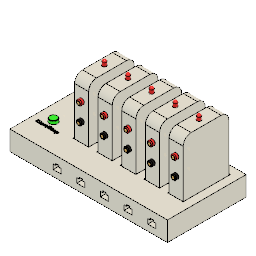
Messbox v3 (Autodesk Fusion 360 design; units mm, degrees)
Autodesk Fusion 360 part; units mm, degrees
sketch "Skizze1" plane through (0, 0, 0) normal (0, 1, 0) x (1, 0, 0)
  line L0 (0, 0) -> (200, 0)
  line L1 (200, 0) -> (200, -100)
  line L2 (200, -100) -> (0, -100)
  line L3 (0, -100) -> (0, 0)
  dimension "d1" = 200
  dimension "d2" = 100
  constraint horizontal L0
  constraint vertical L1
  constraint horizontal L2
  constraint vertical L3
  constraint coincident L0.start L3.end
  measures "d1" distance of L0.start L0.end
  measures "d2" distance of L0.end L1.end
  measures "d91" distance of L0.start
extrude "Extrusion1" add sketch "Skizze1" along normal blind 25
sketch "Skizze2" plane through (0, 25, 0) normal (0, 1, 0) x (-1, 0, 0)
  line L0 (0, 100) -> (-200, 100)
  line L1 (-200, 100) -> (-200, 0)
  line L2 (-200, 0) -> (0, 0)
  line L3 (0, 0) -> (0, 100)
  line L4 (-170, 10) -> (-190, 10)
  line L5 (-190, 10) -> (-190, 70)
  line L6 (-190, 70) -> (-170, 70)
  line L7 (-170, 70) -> (-170, 10)
  line L8 (-140, 10) -> (-160, 10)
  line L9 (-160, 10) -> (-160, 70)
  line L10 (-160, 70) -> (-140, 70)
  line L11 (-140, 70) -> (-140, 10)
  line L12 (-110, 10) -> (-130, 10)
  line L13 (-130, 10) -> (-130, 70)
  line L14 (-130, 70) -> (-110, 70)
  line L15 (-110, 70) -> (-110, 10)
  line L16 (-80, 10) -> (-100, 10)
  line L17 (-100, 10) -> (-100, 70)
  line L18 (-100, 70) -> (-80, 70)
  line L19 (-80, 70) -> (-80, 10)
  line L20 (-100, 10) -> (-110, 10) construction
  line L21 (-130, 10) -> (-140, 10) construction
  line L22 (-160, 10) -> (-170, 10) construction
  line L23 (-70, 10) -> (-50, 10)
  line L24 (-50, 10) -> (-50, 70)
  line L25 (-50, 70) -> (-70, 70)
  line L26 (-70, 70) -> (-70, 10)
  line L27 (-70, 10) -> (-80, 10) construction
  dimension "d5" = 10
  dimension "d6" = 10
  dimension "d8" = 20
  dimension "d38" = 50
  dimension "d162" = 60
  constraint horizontal L4
  constraint vertical L5
  constraint horizontal L6
  constraint vertical L7
  constraint horizontal L8
  constraint vertical L9
  constraint horizontal L10
  constraint vertical L11
  constraint horizontal L12
  constraint vertical L13
  constraint horizontal L14
  constraint vertical L15
  constraint horizontal L16
  constraint vertical L17
  constraint horizontal L18
  constraint vertical L19
  constraint equal L12 L16
  constraint equal L8 L12
  constraint equal L4 L8
  constraint perpendicular L15 L20
  constraint perpendicular L11 L21
  constraint perpendicular L7 L22
  constraint equal L20 L21
  constraint equal L21 L22
  constraint horizontal L13.end L17.end
  constraint horizontal L9.end L13.end
  constraint horizontal L5.end L9.end
  constraint horizontal L23
  constraint vertical L24
  constraint horizontal L25
  constraint vertical L26
  constraint horizontal L27
  constraint horizontal L17.end L25.end
  constraint equal L20 L27
  constraint equal L16 L23
  measures "d5" vertical distance of L1.end L4.end
  measures "d6" horizontal distance of L1.end L4.end
  measures "d8" distance of L4.start L4.end
  measures "d38" horizontal distance of L2.end L23.end
  measures "d162" distance of L4.end L5.end
extrude "Extrusion2" cut sketch "Skizze2" against normal blind 20 contours L4 L5 L6 L7 | L8 L9 L10 L11 | L12 L13 L14 L15 | L16 L17 L18 L19 | L23 L24 L25 L26
sketch "Skizze3" plane through (0, 5, 0) normal (0, 1, 0) x (-1, 0, 0)
  line L0 (-80, 70) -> (-100, 70)
  line L1 (-100, 70) -> (-100, 10)
  line L2 (-100, 10) -> (-80, 10)
  line L3 (-80, 10) -> (-80, 70)
  line L4 (-81, 11) -> (-99, 11)
  line L5 (-99, 11) -> (-99, 69)
  line L6 (-99, 69) -> (-81, 69)
  line L7 (-81, 69) -> (-81, 11)
  line L8 (-111, 11) -> (-129, 11)
  line L9 (-129, 11) -> (-129, 69)
  line L10 (-129, 69) -> (-111, 69)
  line L11 (-111, 69) -> (-111, 11)
  line L12 (-141, 11) -> (-159, 11)
  line L13 (-159, 11) -> (-159, 69)
  line L14 (-159, 69) -> (-141, 69)
  line L15 (-141, 69) -> (-141, 11)
  line L16 (-171, 11) -> (-189, 11)
  line L17 (-189, 11) -> (-189, 69)
  line L18 (-189, 69) -> (-171, 69)
  line L19 (-171, 69) -> (-171, 11)
  line L20 (-51, 11) -> (-69, 11)
  line L21 (-69, 11) -> (-69, 69)
  line L22 (-69, 69) -> (-51, 69)
  line L23 (-51, 69) -> (-51, 11)
  point P0 (-110, 10)
  point P1 (-130, 10)
  point P2 (-130, 70)
  point P3 (-110, 70)
  point P4 (-140, 10)
  point P5 (-160, 10)
  point P6 (-160, 70)
  point P7 (-140, 70)
  point P8 (-170, 10)
  point P9 (-190, 10)
  point P10 (-190, 70)
  point P11 (-70, 10)
  point P12 (-50, 70)
  dimension "d12" = 1
  dimension "d13" = 1
  dimension "d14" = 1
  dimension "d15" = 1
  dimension "d16" = 1
  dimension "d17" = 1
  dimension "d18" = 1
  dimension "d19" = 1
  dimension "d20" = 1
  dimension "d21" = 1
  dimension "d22" = 1
  dimension "d23" = 1
  dimension "d24" = 1
  dimension "d25" = 1
  dimension "d26" = 1
  dimension "d27" = 1
  dimension "d39" = 1
  dimension "d40" = 1
  dimension "d41" = 1
  dimension "d42" = 1
  constraint horizontal L4
  constraint vertical L5
  constraint horizontal L6
  constraint vertical L7
  constraint horizontal L8
  constraint vertical L9
  constraint horizontal L10
  constraint vertical L11
  constraint horizontal L12
  constraint vertical L13
  constraint horizontal L14
  constraint vertical L15
  constraint horizontal L16
  constraint vertical L17
  constraint horizontal L18
  constraint vertical L19
  constraint horizontal L20
  constraint vertical L21
  constraint horizontal L22
  constraint vertical L23
  measures "d12" horizontal distance of L2.end L4.start
  measures "d13" horizontal distance of L1.end L4.end
  measures "d14" vertical distance of L1.end L4.end
  measures "d15" vertical distance of L0.end L5.end
  measures "d16" horizontal distance of L8.start P0
  measures "d17" vertical distance of L8.end P1
  measures "d18" horizontal distance of L9.end P2
  measures "d19" vertical distance of L10.end P3
  measures "d20" horizontal distance of L12.start P4
  measures "d21" vertical distance of L12.end P5
  measures "d22" horizontal distance of L13.end P6
  measures "d23" vertical distance of L14.end P7
  measures "d24" horizontal distance of L16.start P8
  measures "d25" horizontal distance of L16.end P9
  measures "d26" vertical distance of L17.end P10
  measures "d27" vertical distance of L16.end P9
  measures "d39" horizontal distance of L20.end P11
  measures "d40" vertical distance of L20.end P11
  measures "d41" vertical distance of L22.end P12
  measures "d42" horizontal distance of L22.end P12
extrude "Extrusion3" add sketch "Skizze3" along normal blind 90 contours L4 L5 L6 L7 | L8 L9 L10 L11 | L12 L13 L14 L15 | L16 L17 L18 L19 | L20 L21 L22 L23
fillet "Abrundung1" radius 10 8 edges at (90, 95, 69) (120, 95, 69) (120, 95, 11) (90, 95, 11) (150, 95, 11) (180, 95, 11) (180, 95, 69) (150, 95, 69)
fillet "Abrundung3" radius 10 2 edges at (60, 95, 11) (60, 95, 69)
sketch "Skizze4" plane through (0, 95, 0) normal (0, 1, 0) x (-1, 0, 0)
  line L0 (-99, 21) -> (-81, 21)
  line L1 (-81, 21) -> (-81, 59)
  line L2 (-81, 59) -> (-99, 59)
  line L3 (-99, 59) -> (-99, 21)
  circle A0 centre (-90, 40) radius 2.5
  circle A1 centre (-120, 40) radius 2.5
  circle A2 centre (-150, 40) radius 2.5
  circle A3 centre (-180, 40) radius 2.5
  line L4 (-81, 21) -> (-99, 59) construction
  line L5 (-129, 21) -> (-111, 21) construction
  line L6 (-111, 21) -> (-111, 59) construction
  line L7 (-111, 59) -> (-129, 59) construction
  line L8 (-129, 59) -> (-129, 21) construction
  line L9 (-141, 59) -> (-159, 59) construction
  line L10 (-159, 59) -> (-159, 21) construction
  line L11 (-159, 21) -> (-141, 21) construction
  line L12 (-141, 21) -> (-141, 59) construction
  line L13 (-171, 59) -> (-189, 59) construction
  line L14 (-189, 59) -> (-189, 21) construction
  line L15 (-189, 21) -> (-171, 21) construction
  line L16 (-171, 21) -> (-171, 59) construction
  line L17 (-111, 21) -> (-129, 59) construction
  line L18 (-141, 21) -> (-159, 59) construction
  line L19 (-171, 21) -> (-189, 59) construction
  line L20 (-51, 59) -> (-69, 59)
  line L21 (-69, 59) -> (-69, 21)
  line L22 (-69, 21) -> (-51, 21)
  line L23 (-51, 21) -> (-51, 59)
  line L24 (-51, 21) -> (-69, 59) construction
  circle A4 centre (-60, 40) radius 2.5
  dimension "d31" = 5
  dimension "d32" = 5
  dimension "d33" = 5
  dimension "d34" = 5
  dimension "d44" = 5
  constraint coincident L0.end L1.start
  constraint coincident L2.end L3.start
  constraint coincident L5.end L6.start
  constraint coincident L7.end L8.start
  constraint coincident L11.end L12.start
  constraint coincident L9.end L10.start
  constraint coincident L15.end L16.start
  constraint coincident L13.end L14.start
  constraint midpoint A0.centre L4
  constraint midpoint A1.centre L17
  constraint midpoint A2.centre L18
  constraint midpoint A3.centre L19
  constraint coincident L22.end L23.start
  constraint coincident L20.end L21.start
  constraint midpoint L24 A4.centre
  measures "d31" diameter of A0
  measures "d32" diameter of A1
  measures "d33" diameter of A2
  measures "d34" diameter of A3
  measures "d44" diameter of A4
extrude "Extrusion4" add sketch "Skizze4" along normal blind 7 contours A0 | A1 | A2 | A3 | A4
fillet "Abrundung2" radius 2.5 4 edges at (92.3308, 102, 39.096) (122.3308, 102, 39.096) (152.3308, 102, 39.096) (182.3308, 102, 39.096)
fillet "Abrundung4" radius 2.5 1 edges at (62.3308, 102, 39.096)
sketch "Skizze5" plane through (0, 95, 0) normal (0, 1, 0) x (-1, 0, 0)
  circle A0 centre (-180, 40) radius 2.5
  line L0 (-171, 59) -> (-189, 59)
  line L1 (-189, 59) -> (-189, 21)
  line L2 (-189, 21) -> (-171, 21)
  line L3 (-171, 21) -> (-171, 59)
  circle A1 centre (-60, 40) radius 2.5
  circle A2 centre (-90, 40) radius 2.5
  circle A3 centre (-120, 40) radius 2.5
  circle A4 centre (-150, 40) radius 2.5
  circle A5 centre (-180, 40) radius 2.5
  circle A6 centre (-60, 40) radius 2.65
  circle A7 centre (-90, 40) radius 2.65
  circle A8 centre (-120, 40) radius 2.65
  circle A9 centre (-150, 40) radius 2.65
  circle A10 centre (-180, 40) radius 2.65
  dimension "d46" = 5.3
  dimension "d47" = 5.3
  dimension "d48" = 5.3
  dimension "d49" = 5.3
  dimension "d50" = 5.3
  constraint concentric A1 A6
  constraint concentric A2 A7
  constraint concentric A3 A8
  constraint concentric A4 A9
  constraint concentric A5 A10
  measures "d46" diameter of A6
  measures "d47" diameter of A7
  measures "d48" diameter of A8
  measures "d49" diameter of A9
  measures "d50" diameter of A10
sketch "Skizze6" plane through (0, 95, 0) normal (0, 1, 0) x (-1, 0, 0)
  circle A0 centre (-120, 40) radius 2.5
  line L0 (-129, 21) -> (-111, 21)
  line L1 (-111, 21) -> (-111, 59)
  line L2 (-111, 59) -> (-129, 59)
  line L3 (-129, 59) -> (-129, 21)
extrude "Extrusion5" cut sketch "Skizze5" against normal blind 5 contours A6 | A7 | A8 | A9 | A10
sketch "Skizze7" plane through (0, 0, 69) normal (0, 0, 1) x (1, 0, 0)
  line L0 (69, 85) -> (51, 85)
  line L1 (51, 85) -> (51, 5)
  line L2 (51, 5) -> (69, 5)
  line L3 (69, 5) -> (69, 85)
  circle A0 centre (60, 70) radius 3.5
  circle A1 centre (90, 70) radius 3.5
  circle A2 centre (120, 70) radius 3.5
  circle A3 centre (150, 70) radius 3.5
  circle A4 centre (180, 70) radius 3.5
  circle A5 centre (60, 48) radius 3.5
  circle A6 centre (90, 48) radius 3.5
  circle A7 centre (120, 48) radius 3.5
  circle A8 centre (150, 48) radius 3.5
  circle A9 centre (180, 48) radius 3.5
  line L4 (51, 85) -> (60, 70) construction
  line L5 (60, 70) -> (69, 85) construction
  line L6 (99, 85) -> (81, 85) construction
  line L7 (81, 85) -> (81, 5) construction
  line L8 (81, 5) -> (99, 5) construction
  line L9 (99, 5) -> (99, 85) construction
  line L10 (129, 85) -> (111, 85) construction
  line L11 (111, 85) -> (111, 5) construction
  line L12 (111, 5) -> (129, 5) construction
  line L13 (129, 5) -> (129, 85) construction
  line L14 (159, 85) -> (141, 85) construction
  line L15 (141, 85) -> (141, 5) construction
  line L16 (141, 5) -> (159, 5) construction
  line L17 (159, 5) -> (159, 85) construction
  line L18 (189, 85) -> (171, 85) construction
  line L19 (171, 85) -> (171, 5) construction
  line L20 (171, 5) -> (189, 5) construction
  line L21 (189, 5) -> (189, 85) construction
  line L22 (81, 85) -> (90, 70) construction
  line L23 (90, 70) -> (99, 85) construction
  line L24 (111, 85) -> (120, 70) construction
  line L25 (120, 70) -> (129, 85) construction
  line L26 (141, 85) -> (150, 70) construction
  line L27 (150, 70) -> (159, 85) construction
  line L28 (171, 85) -> (180, 70) construction
  line L29 (180, 70) -> (189, 85) construction
  dimension "d53" = 7
  dimension "d54" = 7
  dimension "d55" = 7
  dimension "d56" = 7
  dimension "d57" = 7
  dimension "d58" = 7
  dimension "d59" = 7
  dimension "d60" = 7
  dimension "d61" = 7
  dimension "d62" = 7
  dimension "d63" = 15
  dimension "d64" = 22
  constraint horizontal A0.centre A1.centre
  constraint horizontal A1.centre A2.centre
  constraint horizontal A2.centre A3.centre
  constraint horizontal A3.centre A4.centre
  constraint horizontal A5.centre A6.centre
  constraint horizontal A6.centre A7.centre
  constraint horizontal A8.centre A9.centre
  constraint horizontal A7.centre A8.centre
  constraint vertical A0.centre A5.centre
  constraint vertical A1.centre A6.centre
  constraint vertical A2.centre A7.centre
  constraint vertical A3.centre A8.centre
  constraint vertical A4.centre A9.centre
  constraint coincident L0.end L1.start
  constraint coincident A0.centre L4.end
  constraint coincident L0.start L3.end
  constraint coincident L6.end L7.start
  constraint coincident A1.centre L22.end
  constraint coincident L6.start L9.end
  constraint coincident L10.end L11.start
  constraint coincident A2.centre L24.end
  constraint coincident L10.start L13.end
  constraint coincident L14.end L15.start
  constraint coincident A3.centre L26.end
  constraint coincident L14.start L17.end
  constraint coincident L18.end L19.start
  constraint coincident A4.centre L28.end
  constraint coincident L18.start L21.end
  constraint equal L4 L5
  constraint equal L22 L23
  constraint equal L24 L25
  constraint equal L26 L27
  constraint equal L28 L29
  measures "d53" diameter of A0
  measures "d54" diameter of A1
  measures "d55" diameter of A2
  measures "d56" diameter of A3
  measures "d57" diameter of A4
  measures "d58" diameter of A5
  measures "d59" diameter of A6
  measures "d60" diameter of A7
  measures "d61" diameter of A8
  measures "d62" diameter of A9
  measures "d63" vertical distance of L0.end A0.centre
  measures "d64" distance of A0.centre A5.centre
extrude "Extrusion6" add sketch "Skizze7" along normal blind 4 contours A0 | A1 | A2 | A3 | A4 | A5 | A6 | A7 | A8 | A9
sketch "Skizze8" plane through (0, 0, 73) normal (0, 0, 1) x (1, 0, 0)
  circle A0 centre (60, 70) radius 3.5
  circle A1 centre (120, 48) radius 3.5
  circle A2 centre (150, 48) radius 3.5
  circle A3 centre (150, 70) radius 3.5
  circle A4 centre (120, 70) radius 3.5
  circle A5 centre (90, 48) radius 3.5
  circle A6 centre (90, 70) radius 3.5
  circle A7 centre (60, 48) radius 3.5
  circle A8 centre (60, 70) radius 3.5
  circle A9 centre (180, 70) radius 3.5
  circle A10 centre (180, 48) radius 3.5
  circle A11 centre (60, 70) radius 2
  circle A12 centre (60, 48) radius 2
  circle A13 centre (90, 70) radius 2
  circle A14 centre (90, 48) radius 2
  circle A15 centre (120, 70) radius 2
  circle A16 centre (120, 48) radius 2
  circle A17 centre (150, 70) radius 2
  circle A18 centre (150, 48) radius 2
  circle A19 centre (180, 70) radius 2
  circle A20 centre (180, 48) radius 2
  point P0 (176.5, 70)
  dimension "d67" = 4
  dimension "d68" = 4
  dimension "d69" = 4
  dimension "d70" = 4
  dimension "d71" = 4
  dimension "d72" = 4
  dimension "d73" = 4
  dimension "d74" = 4
  dimension "d75" = 4
  dimension "d76" = 4
  constraint concentric A0 A11
  constraint concentric A7 A12
  constraint concentric A6 A13
  constraint concentric A5 A14
  constraint concentric A4 A15
  constraint concentric A1 A16
  constraint concentric A3 A17
  constraint concentric A2 A18
  constraint concentric A9 A19
  constraint concentric A10 A20
  measures "d67" diameter of A11
  measures "d68" diameter of A12
  measures "d69" diameter of A13
  measures "d70" diameter of A14
  measures "d71" diameter of A15
  measures "d72" diameter of A16
  measures "d73" diameter of A17
  measures "d74" diameter of A18
  measures "d75" diameter of A19
  measures "d76" diameter of A20
extrude "Extrusion7" cut sketch "Skizze8" against normal blind 20 contours A11 | A12 | A13 | A14 | A15 | A16 | A17 | A18 | A19 | A20
fillet "Abrundung5" radius 1 10 edges at (56.7369, 68.7343, 73) (56.7369, 46.7343, 73) (86.7369, 46.7343, 73) (86.7369, 68.7343, 73) (116.7369, 68.7343, 73) (116.7369, 46.7343, 73) (146.7369, 68.7343, 73) (146.7369, 46.7343, 73) (176.7369, 68.7343, 73) (176.7369, 46.7343, 73)
sketch "Skizze9" plane through (0, 0, 0) normal (-1, 0, 0) x (0, 0, 1)
  line L0 (0, 0) -> (100, 0)
  line L1 (100, 0) -> (100, 25)
  line L2 (100, 25) -> (0, 25)
  line L3 (0, 25) -> (0, 0)
  line L4 (25.4, 8.1539) -> (34.4, 8.1539)
  line L5 (34.4, 8.1539) -> (34.4, 4.1539)
  line L6 (34.4, 4.1539) -> (25.4, 4.1539)
  line L7 (25.4, 4.1539) -> (25.4, 8.1539)
  line L8 (54.9, 7.1539) -> (62.9, 7.1539)
  line L9 (62.9, 7.1539) -> (62.9, 4.1539)
  line L10 (62.9, 4.1539) -> (54.9, 4.1539)
  line L11 (54.9, 4.1539) -> (54.9, 7.1539)
  line L12 (67.5, 7.1539) -> (75.5, 7.1539)
  line L13 (75.5, 7.1539) -> (75.5, 4.1539)
  line L14 (75.5, 4.1539) -> (67.5, 4.1539)
  line L15 (67.5, 4.1539) -> (67.5, 7.1539)
  line L16 (0, 0) -> (17.5, 0) construction
  line L17 (82.5, 0) -> (100, 0) construction
  point P0 (29.9, 4.1539)
  point P1 (58.9, 4.1539)
  point P2 (71.5, 4.1539)
  point P3 (17.5, 0)
  point P4 (82.5, 0)
  dimension "d80" = 9
  dimension "d81" = 4
  dimension "d82" = 8
  dimension "d83" = 8
  dimension "d84" = 3
  dimension "d85" = 3
  dimension "d88" = 12.4
  dimension "d90" = 41.4
  dimension "d91" = 54
  dimension "d92" = 65
  constraint horizontal L4
  constraint vertical L5
  constraint horizontal L6
  constraint vertical L7
  constraint horizontal L8
  constraint vertical L9
  constraint horizontal L10
  constraint vertical L11
  constraint horizontal L12
  constraint vertical L13
  constraint horizontal L14
  constraint vertical L15
  constraint horizontal L5.end L10.end
  constraint horizontal L10.end L14.end
  constraint midpoint L6 P0
  constraint midpoint L10 P1
  constraint midpoint L14 P2
  constraint coincident L0 P3
  constraint coincident L0 P4
  constraint coincident L0.start L3.end
  constraint coincident P3 L16.end
  constraint coincident P4 L17.start
  constraint coincident L0.end L1.start
  constraint equal L16 L17
  measures "d80" distance of L4.start L4.end
  measures "d81" distance of L4.start L6.end
  measures "d82" distance of L8.start L8.end
  measures "d83" distance of L12.start L12.end
  measures "d84" distance of L12.start L14.end
  measures "d85" distance of L8.start L10.end
  measures "d88" horizontal distance of P0 P3
  measures "d90" horizontal distance of P1 P3
  measures "d91" horizontal distance of P2 P3
  measures "d92" distance of P3 P4
extrude "Extrusion8" cut sketch "Skizze9" against normal blind 5 contours L4 L5 L6 L7 | L8 L9 L10 L11 | L12 L13 L14 L15
sketch "Skizze10" plane through (5, 0, 0) normal (-1, 0, 0) x (0, 0, 1)
  line L0 (25.4, 4.1539) -> (34.4, 4.1539)
  line L1 (34.4, 4.1539) -> (34.4, 8.1539)
  line L2 (34.4, 8.1539) -> (25.4, 8.1539)
  line L3 (25.4, 8.1539) -> (25.4, 4.1539)
  line L4 (26.7, 7.6539) -> (33.1, 7.6539)
  line L5 (33.1, 7.6539) -> (33.1, 5.8539)
  line L6 (33.1, 5.8539) -> (32.1, 4.8539)
  line L7 (32.1, 4.8539) -> (27.7, 4.8539)
  line L8 (27.7, 4.8539) -> (26.7, 5.8539)
  line L9 (26.7, 5.8539) -> (26.7, 7.6539)
  line L10 (25.4, 8.1539) -> (26.7, 7.6539) construction
  line L11 (33.1, 7.6539) -> (34.4, 8.1539) construction
  dimension "d95" = 6.4
  dimension "d96" = 2.8
  dimension "d97" = 135
  dimension "d98" = 1
  dimension "d99" = 0.5
  constraint parallel L2 L4
  constraint perpendicular L4 L5
  constraint parallel L4 L7
  constraint vertical L9
  constraint equal L6 L8
  constraint equal L5 L9
  constraint coincident L2.end L3.start
  constraint coincident L1.end L2.start
  constraint equal L10 L11
  measures "d95" distance of L4.start L4.end
  measures "d96" vertical distance of L4.start L7.end
  measures "d97" angle of L7 L8
  measures "d98" horizontal distance of L7.end L8.end
  measures "d99" vertical distance of L4.start L2.end
extrude "Extrusion9" add sketch "Skizze10" along normal blind 4 contours L4 L5 L6 L7 L8 L9
sketch "Skizze11" plane through (1, 0, 0) normal (-1, 0, 0) x (0, 0, 1)
  line L0 (26.7, 5.8539) -> (27.7, 4.8539)
  line L1 (27.7, 4.8539) -> (32.1, 4.8539)
  line L2 (32.1, 4.8539) -> (33.1, 5.8539)
  line L3 (33.1, 5.8539) -> (33.1, 7.6539)
  line L4 (33.1, 7.6539) -> (26.7, 7.6539)
  line L5 (26.7, 7.6539) -> (26.7, 5.8539)
  line L6 (27, 7.3539) -> (32.8, 7.3539)
  line L7 (32.8, 7.3539) -> (32.8, 5.9782)
  line L8 (32.8, 5.9782) -> (31.9757, 5.1539)
  line L9 (31.9757, 5.1539) -> (27.8243, 5.1539)
  line L10 (27.8243, 5.1539) -> (27, 5.9782)
  line L11 (27, 5.9782) -> (27, 7.3539)
  line L12 (32.6, 5.3539) -> (32.3879, 5.566) construction
  line L13 (27.2, 5.3539) -> (27.4121, 5.566) construction
  line L14 (27.75, 6.6539) -> (32.05, 6.6539)
  line L15 (32.05, 6.6539) -> (31.55, 6.1539)
  line L16 (31.55, 6.1539) -> (28.25, 6.1539)
  line L17 (28.25, 6.1539) -> (27.75, 6.6539)
  line L18 (29.9, 6.6539) -> (29.9, 7.3539) construction
  dimension "d102" = 0.3
  dimension "d103" = 0.3
  dimension "d104" = 0.3
  dimension "d105" = 0.3
  dimension "d107" = 0.3
  dimension "d108" = 0.3
  dimension "d109" = 0.5
  dimension "d110" = 135
  dimension "d111" = 3.3
  dimension "d112" = 0.7
  constraint horizontal L6
  constraint perpendicular L6 L7
  constraint parallel L6 L9
  constraint perpendicular L8 L10
  constraint vertical L11
  constraint parallel L0 L10
  constraint midpoint L2 L12.start
  constraint midpoint L8 L12.end
  constraint midpoint L0 L13.start
  constraint midpoint L10 L13.end
  constraint perpendicular L3 L14
  constraint perpendicular L3 L16
  constraint equal L15 L17
  constraint midpoint L14 L18.start
  constraint coincident L6 L18.end
  constraint perpendicular L6 L18
  constraint midpoint L6 L18.end
  measures "d102" horizontal distance of L3.end L6.end
  measures "d103" vertical distance of L3.end L6.end
  measures "d104" horizontal distance of L4.end L6.start
  measures "d105" vertical distance of L0.end L9.end
  measures "d107" distance of L13.start L13.end
  measures "d108" distance of L12.start L12.end
  measures "d109" vertical distance of L14.start L16.end
  measures "d110" angle of L15 L16
  measures "d111" distance of L15.end L16.end
  measures "d112" vertical distance of L6.start L14.start
extrude "Extrusion10" cut sketch "Skizze11" against normal blind 4 contours L6 L7 L8 L9 L10 L11
sketch "Skizze12" plane through (5, 0, 0) normal (-1, 0, 0) x (0, 0, 1)
  line L0 (54.9, 4.1539) -> (62.9, 4.1539)
  line L1 (62.9, 4.1539) -> (62.9, 7.1539)
  line L2 (62.9, 7.1539) -> (54.9, 7.1539)
  line L3 (54.9, 7.1539) -> (54.9, 4.1539)
  line L4 (55.475, 6.5539) -> (62.325, 6.5539)
  line L5 (62.325, 6.5539) -> (62.325, 5.5539)
  line L6 (62.325, 5.5539) -> (61.525, 4.7539)
  line L7 (61.525, 4.7539) -> (56.275, 4.7539)
  line L8 (56.275, 4.7539) -> (55.475, 5.5539)
  line L9 (55.475, 5.5539) -> (55.475, 6.5539)
  line L10 (58.9, 6.5539) -> (58.9, 7.1539) construction
  line L11 (68.075, 6.5539) -> (74.925, 6.5539)
  line L12 (74.925, 6.5539) -> (74.925, 5.5539)
  line L13 (74.925, 5.5539) -> (74.125, 4.7539)
  line L14 (74.125, 4.7539) -> (68.875, 4.7539)
  line L15 (68.875, 4.7539) -> (68.075, 5.5539)
  line L16 (68.075, 5.5539) -> (68.075, 6.5539)
  line L17 (67.5, 7.1539) -> (75.5, 7.1539) construction
  line L18 (67.5, 4.1539) -> (67.5, 7.1539) construction
  line L19 (75.5, 4.1539) -> (67.5, 4.1539) construction
  line L20 (75.5, 7.1539) -> (75.5, 4.1539) construction
  line L21 (71.5, 6.5539) -> (71.5, 7.1539) construction
  dimension "d115" = 6.85
  dimension "d116" = 1.8
  dimension "d117" = 135
  dimension "d118" = 1
  dimension "d119" = 135
  dimension "d120" = 1
  dimension "d121" = 6.85
  dimension "d122" = 1.8
  dimension "d123" = 0.6
  dimension "d124" = 0.6
  constraint perpendicular L1 L4
  constraint perpendicular L4 L5
  constraint perpendicular L5 L7
  constraint vertical L9
  constraint equal L6 L8
  constraint equal L5 L9
  constraint midpoint L4 L10.start
  constraint midpoint L2 L10.end
  constraint vertical L10
  constraint horizontal L11
  constraint perpendicular L11 L12
  constraint perpendicular L12 L14
  constraint perpendicular L13 L15
  constraint vertical L16
  constraint equal L13 L15
  constraint midpoint L11 L21.start
  constraint midpoint L17 L21.end
  constraint vertical L21
  measures "d115" distance of L4.start L4.end
  measures "d116" vertical distance of L4.start L7.end
  measures "d117" angle of L6 L7
  measures "d118" distance of L4.end L5.end
  measures "d119" angle of L13 L14
  measures "d120" distance of L11.end L12.end
  measures "d121" distance of L11.start L11.end
  measures "d122" vertical distance of L11.start L14.end
  measures "d123" vertical distance of L2.end L4.start
  measures "d124" vertical distance of L11.start L17.start
extrude "Extrusion11" add sketch "Skizze12" along normal blind 4 contours L4 L5 L6 L7 L8 L9 | L11 L12 L13 L14 L15 L16
sketch "Skizze13" plane through (1, 0, 0) normal (-1, 0, 0) x (0, 0, 1)
  line L0 (68.075, 5.5539) -> (68.875, 4.7539)
  line L1 (68.875, 4.7539) -> (74.125, 4.7539)
  line L2 (74.125, 4.7539) -> (74.925, 5.5539)
  line L3 (74.925, 5.5539) -> (74.925, 6.5539)
  line L4 (74.925, 6.5539) -> (68.075, 6.5539)
  line L5 (68.075, 6.5539) -> (68.075, 5.5539)
  line L6 (68.375, 5.6782) -> (74.625, 5.6782)
  line L7 (74.625, 5.6782) -> (74.0007, 5.0539)
  line L8 (74.0007, 5.0539) -> (68.9993, 5.0539)
  line L9 (68.9993, 5.0539) -> (68.375, 5.6782)
  line L10 (62.025, 5.6782) -> (61.4007, 5.0539)
  line L11 (61.4007, 5.0539) -> (56.3993, 5.0539)
  line L12 (56.3993, 5.0539) -> (55.775, 5.6782)
  line L13 (55.775, 5.6782) -> (62.025, 5.6782)
  line L14 (69.0629, 0.116) -> (69.275, -0.0961) construction
  line L15 (61.525, 4.7539) -> (62.325, 5.5539) construction
  line L16 (56.6463, 0.2995) -> (56.8585, 0.0874) construction
  point P0 (56.275, 4.7539)
  point P1 (55.475, 6.5539)
  point P2 (62.325, 6.5539)
  dimension "d127" = 0.3
  dimension "d128" = 0.3
  dimension "d129" = 0.3
  dimension "d130" = 0.3
  dimension "d131" = 0.3
  dimension "d132" = 0.3
  dimension "d135" = 0.3
  dimension "d136" = 0.3
  constraint parallel L4 L6
  constraint parallel L6 L8
  constraint perpendicular L0 L10
  constraint parallel L8 L11
  constraint perpendicular L10 L12
  constraint parallel L11 L13
  constraint parallel L2 L7
  constraint parallel L0 L9
  constraint coincident L7 L14.start
  constraint coincident L2 L14.end
  constraint perpendicular L2 L14
  constraint coincident L10 L16.start
  constraint coincident L15 L16.end
  constraint perpendicular L15 L16
  measures "d127" vertical distance of L11.end P0
  measures "d128" horizontal distance of L12.end P1
  measures "d129" horizontal distance of L10.start P2
  measures "d130" vertical distance of L0.end L8.end
  measures "d131" horizontal distance of L4.end L6.start
  measures "d132" horizontal distance of L3.end L6.end
  measures "d135" distance of L16.start L16.end
  measures "d136" distance of L14.start L14.end
extrude "Extrusion12" cut sketch "Skizze13" against normal blind 4 contours L6 L7 L8 L9 | L10 L11 L12 L13
sketch "Skizze14" plane through (0, 25, 0) normal (0, 1, 0) x (-1, 0, 0)
  line L0 (-160, 10) -> (-160, 70)
  line L1 (-160, 70) -> (-140, 70)
  line L2 (-140, 70) -> (-140, 10)
  line L3 (-140, 10) -> (-160, 10)
  line L4 (-100, 10) -> (-100, 70)
  line L5 (-100, 70) -> (-80, 70)
  line L6 (-80, 70) -> (-80, 10)
  line L7 (-80, 10) -> (-100, 10)
  line L8 (-190, 10) -> (-190, 70)
  line L9 (-190, 70) -> (-170, 70)
  line L10 (-170, 70) -> (-170, 10)
  line L11 (-170, 10) -> (-190, 10)
  line L12 (-130, 10) -> (-130, 70)
  line L13 (-130, 70) -> (-110, 70)
  line L14 (-110, 70) -> (-110, 10)
  line L15 (-110, 10) -> (-130, 10)
  line L16 (-50, 10) -> (-70, 10)
  line L17 (-70, 10) -> (-70, 70)
  line L18 (-70, 70) -> (-50, 70)
  line L19 (-50, 70) -> (-50, 10)
  line L20 (0, 100) -> (-200, 100)
  line L21 (-200, 100) -> (-200, 0)
  line L22 (-200, 0) -> (0, 0)
  line L23 (0, 0) -> (0, 100)
  circle A0 centre (-19.3652, 63.9359) radius 5
  dimension "d139" = 10
  measures "d139" diameter of A0
extrude "Extrusion13" add sketch "Skizze14" along normal blind 4 contours A0
sketch "Skizze15" plane through (0, 25, 0) normal (0, 1, 0) x (-1, 0, 0)
  circle A0 centre (-19.3652, 63.9359) radius 5
  line L0 (-160, 10) -> (-160, 70)
  line L1 (-160, 70) -> (-140, 70)
  line L2 (-140, 70) -> (-140, 10)
  line L3 (-140, 10) -> (-160, 10)
  line L4 (-100, 10) -> (-100, 70)
  line L5 (-100, 70) -> (-80, 70)
  line L6 (-80, 70) -> (-80, 10)
  line L7 (-80, 10) -> (-100, 10)
  line L8 (-190, 10) -> (-190, 70)
  line L9 (-190, 70) -> (-170, 70)
  line L10 (-170, 70) -> (-170, 10)
  line L11 (-170, 10) -> (-190, 10)
  line L12 (-130, 10) -> (-130, 70)
  line L13 (-130, 70) -> (-110, 70)
  line L14 (-110, 70) -> (-110, 10)
  line L15 (-110, 10) -> (-130, 10)
  line L16 (-50, 10) -> (-70, 10)
  line L17 (-70, 10) -> (-70, 70)
  line L18 (-70, 70) -> (-50, 70)
  line L19 (-50, 70) -> (-50, 10)
  line L20 (0, 100) -> (-200, 100)
  line L21 (-200, 100) -> (-200, 0)
  line L22 (-200, 0) -> (0, 0)
  line L23 (0, 0) -> (0, 100)
  circle A1 centre (-19.3652, 63.9359) radius 5.15
  dimension "d142" = 10.3
  constraint concentric A0 A1
  measures "d142" diameter of A1
extrude "Extrusion14" cut sketch "Skizze15" against normal blind 5 contours A1
fillet "Abrundung6" radius 0.5 1 edges at (24.0269, 29, 62.1278)
sketch "Skizze16" plane through (0, 25, 0) normal (0, 1, 0) x (-1, 0, 0)
  circle A0 centre (-19.3652, 63.9359) radius 5.15
  line L0 (-160, 10) -> (-160, 70)
  line L1 (-160, 70) -> (-140, 70)
  line L2 (-140, 70) -> (-140, 10)
  line L3 (-140, 10) -> (-160, 10)
  line L4 (-100, 10) -> (-100, 70)
  line L5 (-100, 70) -> (-80, 70)
  line L6 (-80, 70) -> (-80, 10)
  line L7 (-80, 10) -> (-100, 10)
  line L8 (-190, 10) -> (-190, 70)
  line L9 (-190, 70) -> (-170, 70)
  line L10 (-170, 70) -> (-170, 10)
  line L11 (-170, 10) -> (-190, 10)
  line L12 (-130, 10) -> (-130, 70)
  line L13 (-130, 70) -> (-110, 70)
  line L14 (-110, 70) -> (-110, 10)
  line L15 (-110, 10) -> (-130, 10)
  line L16 (-50, 10) -> (-70, 10)
  line L17 (-70, 10) -> (-70, 70)
  line L18 (-70, 70) -> (-50, 70)
  line L19 (-50, 70) -> (-50, 10)
  line L20 (0, 100) -> (-200, 100)
  line L21 (-200, 100) -> (-200, 0)
  line L22 (-200, 0) -> (0, 0)
  line L23 (0, 0) -> (0, 100)
  line L24 (-7.2882, 76.7519) -> (-35.5157, 76.7519) construction
  line L25 (-35.5157, 76.7519) -> (-35.5157, 70.7519) construction
  line L26 (-35.5157, 70.7519) -> (-7.2882, 70.7519) construction
  line L27 (-7.2882, 70.7519) -> (-7.2882, 76.7519) construction
  text T0 "Start/Stop" font "Arial" height 6 bold align ink ink in box 0 x 0 at (-7.2982, 76.7319) x (-1, 0) y (0, -1) spacing 1 height is em
  constraint perpendicular L24 L25
  constraint parallel L24 L26
  constraint parallel L25 L27
sketch "Skizze17" plane through (189, 0, 0) normal (1, 0, 0) x (0, 0, -1)
  arc A0 (-59, 95) -> (-69, 85) centre (-59, 85) ccw
  line L0 (-69, 85) -> (-69, 5)
  line L1 (-69, 5) -> (-11, 5)
  line L2 (-11, 5) -> (-11, 85)
  arc A1 (-11, 85) -> (-21, 95) centre (-21, 85) ccw
  line L3 (-21, 95) -> (-59, 95)
sketch "Skizze18" plane through (51, 0, 0) normal (-1, 0, 0) x (0, 0, 1)
  arc A0 (69, 85) -> (59, 95) centre (59, 85) ccw
  line L0 (59, 95) -> (21, 95)
  arc A1 (21, 95) -> (11, 85) centre (21, 85) ccw
  line L1 (11, 85) -> (11, 5)
  line L2 (11, 5) -> (69, 5)
  line L3 (69, 5) -> (69, 85)
  line L4 (24.5601, 71.9399) -> (55.815, 71.9399) construction
  line L5 (55.815, 71.9399) -> (55.815, 81.9399) construction
  line L6 (55.815, 81.9399) -> (24.5601, 81.9399) construction
  line L7 (24.5601, 81.9399) -> (24.5601, 71.9399) construction
  line L8 (15.852, 57.532) -> (64.2749, 57.532) construction
  line L9 (64.2749, 57.532) -> (64.2749, 67.532) construction
  line L10 (64.2749, 67.532) -> (15.852, 67.532) construction
  line L11 (15.852, 67.532) -> (15.852, 57.532) construction
  text T0 "STM32" font "Arial" height 10 align ink ink in box 0 x 0 at (24.5701, 71.9599) x (1, 0) y (0, 1) spacing 1 height is em
  text T1 "+ ext. RAM" font "Arial" height 10 align ink ink in box 0 x 0 at (15.862, 57.552) x (1, 0) y (0, 1) spacing 1 height is em
  constraint perpendicular L4 L5
  constraint parallel L4 L6
  constraint parallel L5 L7
  constraint perpendicular L8 L9
  constraint parallel L8 L10
  constraint parallel L9 L11
sketch "Skizze19" plane through (100, 25, 40) normal (0, 1, 0) x (-1, 0, 0)
sketch "Skizze20" plane through (0, 0, 0) normal (-1, 0, 0) x (0, 0, 1)
  line L0 (34.4, 8.1539) -> (34.4, 4.1539)
  line L1 (34.4, 4.1539) -> (25.4, 4.1539)
  line L2 (25.4, 4.1539) -> (25.4, 8.1539)
  line L3 (25.4, 8.1539) -> (34.4, 8.1539)
  line L4 (62.9, 7.1539) -> (62.9, 4.1539)
  line L5 (62.9, 4.1539) -> (54.9, 4.1539)
  line L6 (54.9, 4.1539) -> (54.9, 7.1539)
  line L7 (54.9, 7.1539) -> (62.9, 7.1539)
  line L8 (75.5, 7.1539) -> (75.5, 4.1539)
  line L9 (75.5, 4.1539) -> (67.5, 4.1539)
  line L10 (67.5, 4.1539) -> (67.5, 7.1539)
  line L11 (67.5, 7.1539) -> (75.5, 7.1539)
  line L12 (0, 0) -> (100, 0)
  line L13 (100, 0) -> (100, 25)
  line L14 (100, 25) -> (0, 25)
  line L15 (0, 25) -> (0, 0)
  line L16 (3.716, 12.3276) -> (75.0481, 12.3276) construction
  line L17 (75.0481, 12.3276) -> (75.0481, 20.3276) construction
  line L18 (75.0481, 20.3276) -> (3.716, 20.3276) construction
  line L19 (3.716, 20.3276) -> (3.716, 12.3276) construction
  text T0 "Raspberry Pi zero w" font "Arial" height 8 align ink ink in box 0 x 0 at (3.726, 12.3476) x (1, 0) y (0, 1) spacing 1 height is em
  constraint perpendicular L16 L17
  constraint parallel L16 L18
  constraint parallel L17 L19
extrude "Extrusion15" add sketch "Skizze18" sketch "Skizze20" along normal blind 0.1 text T1 T0 of sketch 2 text T0
extrude "Extrusion16" add sketch "Skizze16" along normal blind 0.1 text T0
sketch "Skizze21" plane through (0, 0, 100) normal (0, 0, 1) x (1, 0, 0)
  line L0 (0, 0) -> (200, 0)
  line L1 (200, 0) -> (200, 25)
  line L2 (200, 25) -> (0, 25)
  line L3 (0, 25) -> (0, 0)
  line L4 (55, 14) -> (65, 14)
  line L5 (65, 14) -> (65, 8)
  line L6 (65, 8) -> (55, 8)
  line L7 (55, 8) -> (55, 14)
  line L8 (85, 14) -> (95, 14)
  line L9 (95, 14) -> (95, 8)
  line L10 (95, 8) -> (85, 8)
  line L11 (85, 8) -> (85, 14)
  line L12 (115, 14) -> (125, 14)
  line L13 (125, 14) -> (125, 8)
  line L14 (125, 8) -> (115, 8)
  line L15 (115, 8) -> (115, 14)
  line L16 (145, 14) -> (155, 14)
  line L17 (155, 14) -> (155, 8)
  line L18 (155, 8) -> (145, 8)
  line L19 (145, 8) -> (145, 14)
  line L20 (175, 14) -> (185, 14)
  line L21 (185, 14) -> (185, 8)
  line L22 (185, 8) -> (175, 8)
  line L23 (175, 8) -> (175, 14)
  line L24 (58, 14) -> (62, 14)
  line L25 (62, 14) -> (62, 16)
  line L26 (62, 16) -> (58, 16)
  line L27 (58, 16) -> (58, 14)
  line L28 (88, 14) -> (92, 14)
  line L29 (92, 14) -> (92, 16)
  line L30 (92, 16) -> (88, 16)
  line L31 (88, 16) -> (88, 14)
  line L32 (118, 14) -> (122, 14)
  line L33 (122, 14) -> (122, 16)
  line L34 (122, 16) -> (118, 16)
  line L35 (118, 16) -> (118, 14)
  line L36 (148, 14) -> (152, 14)
  line L37 (152, 14) -> (152, 16)
  line L38 (152, 16) -> (148, 16)
  line L39 (148, 16) -> (148, 14)
  line L40 (178, 14) -> (182, 14)
  line L41 (182, 14) -> (182, 16)
  line L42 (182, 16) -> (178, 16)
  line L43 (178, 16) -> (178, 14)
  line L44 (55, 14) -> (58, 14) construction
  line L45 (85, 14) -> (88, 14) construction
  line L46 (115, 14) -> (118, 14) construction
  line L47 (145, 14) -> (148, 14) construction
  line L48 (175, 14) -> (178, 14) construction
  line L49 (65, 8) -> (85, 8) construction
  line L50 (95, 8) -> (115, 8) construction
  line L51 (125, 8) -> (145, 8) construction
  line L52 (155, 8) -> (175, 8) construction
  circle A0 centre (180, 70) radius 3.5 construction
  circle A1 centre (180, 48) radius 3.5 construction
  line L53 (189, 85) -> (171, 85) construction
  line L54 (171, 85) -> (171, 5) construction
  line L55 (171, 5) -> (189, 5) construction
  line L56 (189, 5) -> (189, 85) construction
  line L57 (0, 25) -> (200, 25) construction
  line L58 (171, 5) -> (175, 8) construction
  line L59 (185, 8) -> (189, 5) construction
  circle A2 centre (60, 48) radius 3.5 construction
  circle A3 centre (60, 70) radius 3.5 construction
  line L60 (69, 85) -> (51, 85) construction
  line L61 (51, 85) -> (51, 5) construction
  line L62 (51, 5) -> (69, 5) construction
  line L63 (69, 5) -> (69, 85) construction
  line L64 (51, 5) -> (55, 8) construction
  line L65 (65, 8) -> (69, 5) construction
  dimension "d150" = 10
  dimension "d151" = 4
  dimension "d152" = 2
  dimension "d153" = 3
  dimension "d154" = 6
  dimension "d155" = 3
  constraint horizontal L4
  constraint vertical L5
  constraint horizontal L6
  constraint vertical L7
  constraint horizontal L8
  constraint vertical L9
  constraint horizontal L10
  constraint vertical L11
  constraint horizontal L12
  constraint vertical L13
  constraint horizontal L14
  constraint vertical L15
  constraint vertical L17
  constraint horizontal L18
  constraint vertical L19
  constraint horizontal L20
  constraint vertical L21
  constraint horizontal L22
  constraint vertical L23
  constraint horizontal L24
  constraint vertical L25
  constraint horizontal L26
  constraint vertical L27
  constraint coincident L4 L24.start
  constraint horizontal L28
  constraint vertical L29
  constraint horizontal L30
  constraint vertical L31
  constraint coincident L8 L28.start
  constraint horizontal L32
  constraint vertical L33
  constraint horizontal L34
  constraint vertical L35
  constraint coincident L12 L32.start
  constraint horizontal L36
  constraint vertical L37
  constraint horizontal L38
  constraint vertical L39
  constraint coincident L16 L36.start
  constraint horizontal L40
  constraint vertical L41
  constraint horizontal L42
  constraint vertical L43
  constraint coincident L20 L40.start
  constraint perpendicular L27 L44
  constraint perpendicular L31 L45
  constraint perpendicular L39 L47
  constraint equal L44 L45
  constraint equal L27 L31
  constraint equal L26 L30
  constraint equal L4 L8
  constraint equal L5 L9
  constraint equal L31 L35
  constraint equal L30 L34
  constraint equal L8 L12
  constraint equal L9 L15
  constraint equal L45 L46
  constraint equal L46 L47
  constraint equal L34 L38
  constraint equal L12 L16
  constraint equal L33 L37
  constraint equal L13 L17
  constraint equal L39 L43
  constraint equal L38 L42
  constraint equal L16 L20
  constraint equal L47 L48
  constraint equal L17 L21
  constraint horizontal L5.end L10.end
  constraint horizontal L10.end L14.end
  constraint horizontal L14.end L18.end
  constraint horizontal L18.end L22.end
  constraint equal L51 L52
  constraint equal L50 L51
  constraint equal L49 L50
  constraint coincident L54.end L55.start
  constraint coincident L55.end L56.start
  constraint equal L58 L59
  constraint coincident L61.end L62.start
  constraint coincident L62.end L63.start
  constraint equal L64 L65
  measures "d150" distance of L5.end L6.end
  measures "d151" distance of L25.end L26.end
  measures "d152" distance of L24.end L25.end
  measures "d153" distance of L4.start L24.start
  measures "d154" distance of L4.end L5.end
  measures "d155" vertical distance of L6.end L61.end
extrude "Extrusion17" cut sketch "Skizze21" against normal blind 10 contours L4 L5 L6 L7 L24 | L8 L9 L10 L11 L28 | L12 L13 L14 L15 L32 | L16 L17 L18 L19 L36 | L20 L21 L22 L23 L40
extrude "Extrusion18" cut sketch "Skizze21" against normal blind 4 contours L4 L24 L25 L26 L27 | L8 L28 L29 L30 L31 | L12 L32 L33 L34 L35 | L16 L36 L37 L38 L39 | L20 L40 L41 L42 L43
chamfer "Fase1" distance 4 distance2 2 5 edges at (60, 16, 96) (90, 16, 96) (120, 16, 96) (150, 16, 96) (180, 16, 96) measured on face at (60.6667, 16, 98.6667) measured on face at (90.6667, 16, 98.6667) measured on face at (120.6667, 16, 98.6667) measured on face at (150.6667, 16, 98.6667) measured on face at (180.6667, 16, 98.6667)
